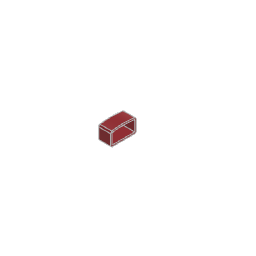
EndCap Closed (Autodesk Fusion 360 design; units mm, degrees)
Autodesk Fusion 360 part; units mm, degrees
sketch "EndCap Profile" plane through (0, -18.7334, 136.7) normal (-1, 0, 0) x (0, 1, 0)
  spline S0 degree 5 poles (18.7334, 131.7635) (18.7472, 131.7725) (18.7754, 131.7914) (18.8198, 131.8224) (18.8833, 131.8692) (18.9694, 131.937) (19.0611, 132.0138) (19.1557, 132.0994) (19.2487, 132.193) (19.3333, 132.2931) (19.4014, 132.398) (19.4456, 132.5057) (19.4603, 132.614) (19.4429, 132.7209) (19.3958, 132.8246) (19.3249, 132.9235) (19.2379, 133.0162) (19.1431, 133.1016) (19.0477, 133.179) (18.9568, 133.2479) (18.873, 133.3082) (18.8128, 133.3496) (18.7716, 133.3768) (18.7458, 133.3932) (18.7334, 133.401) knots 0 0 0 0 0 0 0.05 0.1 0.15 0.2 0.25 0.3 0.35 0.4 0.45 0.5 0.55 0.6 0.65 0.7 0.75 0.8 0.85 0.9 0.95 1 1 1 1 1 1
  line L0 (18.7334, 131.7635) -> (18.7334, 130.1038) construction
  spline S1 degree 5 poles (18.7334, 130.1038) (18.733, 130.0969) (18.734, 130.0831) (18.7414, 130.0625) (18.7627, 130.0353) (18.8083, 130.0019) (18.8718, 129.9701) (18.9509, 129.9418) (19.041, 129.9202) (19.1361, 129.9097) (19.2296, 129.9146) (19.3155, 129.9383) (19.3895, 129.9828) (19.4498, 130.0468) (19.498, 130.1261) (19.5376, 130.2149) (19.5732, 130.3068) (19.6091, 130.3956) (19.649, 130.4771) (19.6945, 130.5496) (19.7461, 130.6131) (19.8031, 130.669) (19.8647, 130.7194) (19.9299, 130.766) (19.9979, 130.8102) (20.0683, 130.8527) (20.1263, 130.8857) (20.1708, 130.9099) (20.2009, 130.9258) (20.216, 130.9336) knots 0 0 0 0 0 0 0.04 0.08 0.12 0.16 0.2 0.24 0.28 0.32 0.36 0.4 0.44 0.48 0.52 0.56 0.6 0.64 0.68 0.72 0.76 0.8 0.84 0.88 0.92 0.96 1 1 1 1 1 1
  line L1 (20.216, 130.9336) -> (20.216, 132.6738) construction
  spline S2 degree 5 poles (20.216, 132.6738) (20.1958, 132.6805) (20.1564, 132.6946) (20.1008, 132.7179) (20.0337, 132.7532) (19.9616, 132.8044) (19.902, 132.8628) (19.8551, 132.9279) (19.8214, 132.9989) (19.8008, 133.0741) (19.7932, 133.1513) (19.7983, 133.2282) (19.8156, 133.3026) (19.8447, 133.3727) (19.885, 133.4375) (19.9358, 133.4966) (19.9847, 133.5392) (20.0258, 133.5684) (20.0551, 133.5868) (20.0703, 133.5957) knots 0 0 0 0 0 0 0.066667 0.133333 0.2 0.266667 0.333333 0.4 0.466667 0.533333 0.6 0.666667 0.733333 0.8 0.866667 0.933333 1 1 1 1 1 1
  line L2 (20.0703, 133.5957) -> (20.878, 133.5957) construction
  spline S3 degree 5 poles (20.878, 133.5957) (20.8852, 133.5982) (20.9, 133.604) (20.9227, 133.6149) (20.9545, 133.634) (20.9962, 133.6655) (21.0392, 133.7047) (21.0818, 133.7513) (21.1214, 133.8055) (21.1541, 133.8667) (21.1761, 133.9344) (21.1843, 134.0073) (21.1764, 134.0832) (21.1526, 134.1593) (21.1148, 134.2318) (21.0661, 134.2975) (21.0101, 134.3539) (20.9503, 134.4004) (20.8895, 134.439) (20.8297, 134.4738) (20.7725, 134.51) (20.7194, 134.5525) (20.6721, 134.6048) (20.633, 134.6679) (20.6049, 134.7405) (20.5907, 134.8196) (20.5931, 134.9019) (20.6146, 134.9836) (20.6568, 135.0624) (20.7206, 135.1364) (20.8067, 135.2047) (20.8934, 135.2545) (20.9684, 135.289) (21.0229, 135.3108) (21.0513, 135.3214) knots 0 0 0 0 0 0 0.033333 0.066667 0.1 0.133333 0.166667 0.2 0.233333 0.266667 0.3 0.333333 0.366667 0.4 0.433333 0.466667 0.5 0.533333 0.566667 0.6 0.633333 0.666667 0.7 0.733333 0.766667 0.8 0.833333 0.866667 0.9 0.933333 0.966667 1 1 1 1 1 1
  line L3 (21.0513, 135.3214) -> (21.0513, 135.7) construction
  line L4 (21.0513, 135.7) -> (33.4156, 135.7) construction
  line L5 (33.4156, 135.7) -> (33.4156, 135.3214) construction
  spline S4 degree 5 poles (33.5888, 133.5957) (33.5816, 133.5982) (33.5669, 133.604) (33.5441, 133.6149) (33.5124, 133.634) (33.4706, 133.6655) (33.4277, 133.7047) (33.385, 133.7513) (33.3455, 133.8055) (33.3128, 133.8667) (33.2907, 133.9344) (33.2826, 134.0073) (33.2904, 134.0832) (33.3142, 134.1593) (33.352, 134.2318) (33.4007, 134.2975) (33.4568, 134.3539) (33.5166, 134.4004) (33.5774, 134.439) (33.6372, 134.4738) (33.6944, 134.51) (33.7475, 134.5525) (33.7947, 134.6048) (33.8338, 134.6679) (33.8619, 134.7405) (33.8762, 134.8196) (33.8738, 134.9019) (33.8523, 134.9836) (33.8101, 135.0624) (33.7462, 135.1364) (33.6601, 135.2047) (33.5734, 135.2545) (33.4984, 135.289) (33.4439, 135.3108) (33.4156, 135.3214) knots 0 0 0 0 0 0 0.033333 0.066667 0.1 0.133333 0.166667 0.2 0.233333 0.266667 0.3 0.333333 0.366667 0.4 0.433333 0.466667 0.5 0.533333 0.566667 0.6 0.633333 0.666667 0.7 0.733333 0.766667 0.8 0.833333 0.866667 0.9 0.933333 0.966667 1 1 1 1 1 1
  line L6 (33.5888, 133.5957) -> (34.3966, 133.5957) construction
  spline S5 degree 5 poles (34.2508, 132.6738) (34.2711, 132.6805) (34.3104, 132.6946) (34.366, 132.7179) (34.4332, 132.7532) (34.5052, 132.8044) (34.5649, 132.8628) (34.6117, 132.9279) (34.6455, 132.9989) (34.666, 133.0741) (34.6736, 133.1513) (34.6685, 133.2282) (34.6512, 133.3026) (34.6221, 133.3727) (34.5819, 133.4375) (34.531, 133.4966) (34.4821, 133.5392) (34.4411, 133.5684) (34.4117, 133.5868) (34.3966, 133.5957) knots 0 0 0 0 0 0 0.066667 0.133333 0.2 0.266667 0.333333 0.4 0.466667 0.533333 0.6 0.666667 0.733333 0.8 0.866667 0.933333 1 1 1 1 1 1
  line L7 (34.2508, 132.6738) -> (34.2508, 130.9336) construction
  spline S6 degree 5 poles (35.7334, 130.1038) (35.7339, 130.0969) (35.7328, 130.0831) (35.7255, 130.0625) (35.7042, 130.0353) (35.6585, 130.0019) (35.595, 129.9701) (35.516, 129.9418) (35.4259, 129.9202) (35.3308, 129.9097) (35.2373, 129.9146) (35.1513, 129.9383) (35.0774, 129.9828) (35.0171, 130.0468) (34.9688, 130.1261) (34.9292, 130.2149) (34.8937, 130.3068) (34.8577, 130.3956) (34.8178, 130.4771) (34.7723, 130.5496) (34.7208, 130.6131) (34.6637, 130.669) (34.6021, 130.7194) (34.537, 130.766) (34.469, 130.8102) (34.3986, 130.8527) (34.3405, 130.8857) (34.296, 130.9099) (34.266, 130.9258) (34.2508, 130.9336) knots 0 0 0 0 0 0 0.04 0.08 0.12 0.16 0.2 0.24 0.28 0.32 0.36 0.4 0.44 0.48 0.52 0.56 0.6 0.64 0.68 0.72 0.76 0.8 0.84 0.88 0.92 0.96 1 1 1 1 1 1
  line L8 (35.7334, 131.7635) -> (35.7334, 130.1038) construction
  spline S7 degree 5 poles (35.7334, 131.7635) (35.7197, 131.7725) (35.6915, 131.7914) (35.6471, 131.8224) (35.5836, 131.8692) (35.4974, 131.937) (35.4057, 132.0138) (35.3111, 132.0994) (35.2181, 132.193) (35.1336, 132.2931) (35.0654, 132.398) (35.0212, 132.5057) (35.0065, 132.614) (35.0239, 132.7209) (35.071, 132.8246) (35.1419, 132.9235) (35.2289, 133.0162) (35.3238, 133.1016) (35.4191, 133.179) (35.51, 133.2479) (35.5938, 133.3082) (35.6541, 133.3496) (35.6953, 133.3768) (35.721, 133.3932) (35.7334, 133.401) knots 0 0 0 0 0 0 0.05 0.1 0.15 0.2 0.25 0.3 0.35 0.4 0.45 0.5 0.55 0.6 0.65 0.7 0.75 0.8 0.85 0.9 0.95 1 1 1 1 1 1
  line L9 (35.7334, 135.7) -> (35.7334, 133.401) construction
  line L10 (35.7334, 135.7) -> (35.7334, 136.7) construction
  line L11 (35.7334, 136.7) -> (18.7334, 136.7) construction
  line L12 (18.7334, 136.7) -> (18.7334, 135.7) construction
  line L13 (18.7334, 135.7) -> (18.7334, 133.401) construction
  line L14 (18.7334, 136.7) -> (35.7334, 136.7)
  line L15 (35.7334, 136.7) -> (35.7334, 128.9)
  line L16 (35.7334, 128.9) -> (18.7334, 128.9)
  line L17 (18.7334, 128.9) -> (18.7334, 136.7)
  arc A0 (18.7334, 128.9) -> (35.7334, 128.9) centre (27.2334, 178.1722) ccw
  line L18 (37.1334, 138.1) -> (37.1334, 127.7346)
  arc A1 (17.3334, 127.7346) -> (37.1334, 127.7346) centre (27.2334, 178.1722) ccw
  line L19 (17.3334, 127.7346) -> (17.3334, 138.1)
  line L20 (17.3334, 138.1) -> (37.1334, 138.1)
  dimension "d121_1" = 7.8
  dimension "d122_1" = -1.4
  dimension "d133_1" = 50
  dimension "d134_1" = 17
  constraint horizontal L14
  constraint vertical L15
  constraint horizontal L16
  constraint vertical L17
  constraint coincident L11.end L12.start
  measures "d121_1" distance of L10.end L15.end
  measures "d133_1" radius of A0
  measures "d134_1" distance of L11.end L10.end
extrude "Extrude1" add sketch "EndCap Profile" along normal blind 10 contours S0 L17 | S0 S7 L14 L15 L16 L17 | L16 A0 | S7 L15 | L18 A1 L19 L20
shell "Shell1" thickness 1.2 removed faces 1 at (0, 7.3939, 2.3402)
sketch "EndCap Hole" plane through (-8.8, 0, 0) normal (1, 0, 0) x (0, 1, 0)
  line L0 (4.85, -1.2) -> (12.15, -1.2)
  line L1 (12.15, -1.2) -> (12.15, -5.6)
  line L2 (12.15, -5.6) -> (4.85, -5.6)
  line L3 (4.85, -5.6) -> (4.85, -1.2)
  arc A0 (17.2, 7.9682) -> (-0.2, 7.9682) centre (8.5, -41.4722) ccw
  line L4 (-0.2, 7.9682) -> (-0.2, -0.2)
  line L5 (-0.2, -0.2) -> (17.2, -0.2)
  line L6 (17.2, -0.2) -> (17.2, 7.9682)
  line L7 (-1.4, -1.4, -1.2) -> (18.4, -1.4, -1.2)
  line L8 (8.5, -0.2) -> (8.5, -1.2) construction
  point P0 (8.5, -1.2)
  point P1 (8.5, -1.2)
  point P2 (8.5, -0.2)
  dimension "d115_1" = 4.4
  dimension "d131_1" = 1
  dimension "d132_1" = 7.3
  constraint horizontal L0
  constraint vertical L1
  constraint horizontal L2
  constraint vertical L3
  constraint midpoint L0 P1
  constraint coincident P1 P0
  constraint midpoint L5 P2
  constraint coincident P2 L8.start
  constraint vertical L8
  measures "d115_1" distance of L0.start L2.end
  measures "d131_1" distance of P2 P1
  measures "d132_1" distance of L1.end L2.end
chamfer "Chamfer1" distance 1 angle 45 8 edges at (-10, 18.4, 3.7827) (-10, 8.5, 9.9278) (-10, -1.4, 3.7827) (-10, 8.5, -1.4) (-5, 18.4, -1.4) (-5, 18.4, 8.9654) (-5, -1.4, -1.4) (-5, -1.4, 8.9654)
named bodies: "End Cap"
